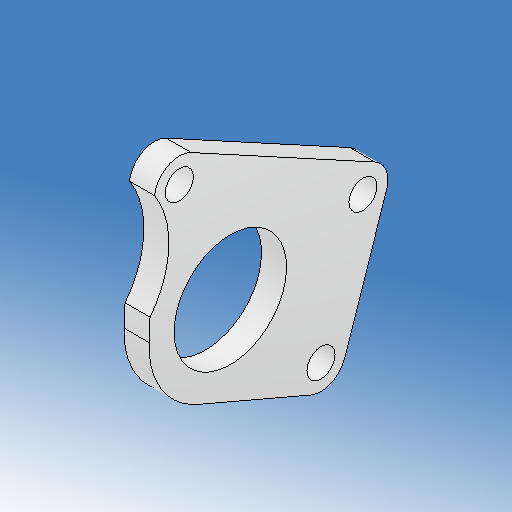
# Autodesk Inventor part: OuterDriveRail
Saved by Autodesk Inventor 2025 (Build 290162000, 162)
## iProperties
Created: 2023-02-06
Part Number: OuterDriveRail
Material: Aluminum 6061
Document SubType Name: Modeling
Designer: kumpu
Density: 2.7 g/cm^3
Appearance: Aluminum - Flat
Mass: 503.524 g
Surface Area: 633.713 cm^2
Volume: 186.49 cm^3
Author: kumpu
Autodesk Inventor part; units mm, degrees
ref_plane "YZ Plane" through (0, 0, 0) normal (1, 0, 0) x (0, 1, 0)
ref_plane "XZ Plane" through (0, 0, 0) normal (0, 1, 0) x (-1, 0, 0)
ref_plane "XY Plane" through (0, 0, 0) normal (0, 0, 1) x (1, 0, 0)
sketch "Sketch1" plane through (0, 0, 0) normal (1, 0, 0) x (0, 1, 0)
  line L0 (111.125, 190.5) -> (36.4799, 190.5)
  line L1 (36.4799, 190.5) -> (-11.1661, 102.5705)
  arc A0 (-11.1661, 102.5705) -> (-11.1661, 90.4695) centre (0, 96.52) ccw
  line L2 (-11.1661, 90.4695) -> (7.6076, 55.8231)
  arc A1 (-11.1661, 6.0505) -> (-11.1661, -6.0505) centre (0, 0) ccw
  line L3 (-11.1661, -6.0505) -> (7.6076, -40.6969)
  arc A2 (-11.1661, -90.4695) -> (-11.1661, -102.5705) centre (0, -96.52) ccw
  line L4 (-11.1661, -102.5705) -> (36.4799, -190.5)
  line L5 (36.4799, -190.5) -> (111.125, -190.5)
  line L6 (111.125, -190.5) -> (111.125, 190.5)
  circle A3 centre (64.6139, -120.5964) radius 6.35 construction
  circle A4 centre (42.5128, -176.727) radius 4.7625 construction
  line L7 (111.125, 0) -> (0, 0) construction
  circle A5 centre (0, 96.52) radius 2.4892 construction
  circle A6 centre (0, 0) radius 2.4892 construction
  circle A7 centre (0, -96.52) radius 2.4892 construction
  line L8 (-11.1661, 6.0505) -> (7.6076, 40.6969)
  arc A8 (7.6076, 40.6969) -> (7.6076, 55.8231) centre (-6.35, 48.26) ccw
  line L9 (-11.1661, -90.4695) -> (7.6076, -55.8231)
  arc A9 (7.6076, -55.8231) -> (7.6076, -40.6969) centre (-6.35, -48.26) ccw
  line L10 (-6.35, -48.26) -> (-6.35, 48.26) construction
  line L11 (-6.35, 0) -> (0, 0) construction
  circle A10 centre (0, 96.52) radius 3.175
  circle A11 centre (0, 0) radius 3.175
  circle A12 centre (0, -96.52) radius 3.175
  circle A13 centre (46.0375, 122.682) radius 3.5687 construction
  circle A14 centre (20.6375, 122.682) radius 3.5687 construction
  circle A15 centre (46.0375, 122.682) radius 3.175
  circle A16 centre (20.6375, 122.682) radius 3.175
  circle A17 centre (100.0125, -94.6341) radius 3.175
  circle A18 centre (74.6125, -94.6341) radius 3.175
  line L12 (0, 96.52) -> (-12.7, 96.52) construction
  circle A19 centre (60.325, -101.6) radius 3.5687 construction
  circle A20 centre (80.899, -155.6385) radius 12.0396 construction
  line L13 (30.099, -178.7242) -> (30.099, -155.6385)
  arc A21 (111.125, -114.8092) -> (30.099, -155.6385) centre (80.899, -155.6385) ccw
  circle A22 centre (60.325, -101.6) radius 3.175
  circle A23 centre (41.275, 177.125) radius 20.6375
  circle A24 centre (41.275, 177.125) radius 26.9875
  circle A25 centre (41.275, 177.125) radius 25.4 construction
  circle A26 centre (85.725, 107.3629) radius 7.9375
  line L14 (-12.7, 190.5) -> (-12.7, -193.5034) construction
  circle A27 centre (85.725, 107.3629) radius 17.78 construction
  circle A28 centre (79.375, 147.5038) radius 22.86 construction
  circle A29 centre (79.375, 147.5038) radius 14.2875
  circle A30 centre (66.675, 254) radius 58.7375 construction
  circle A31 centre (66.675, -254) radius 58.7375 construction
  circle A32 centre (80.899, -155.6385) radius 47.527 construction
  circle A33 centre (100.0125, -94.6341) radius 6.35 construction
  circle A34 centre (74.6125, -94.6341) radius 6.35 construction
  circle A35 centre (17.4625, -131.1466) radius 3.175
  circle A36 centre (17.4625, -131.1466) radius 6.35 construction
  line L15 (9.525, 127) -> (-15.875, 127) construction
  line L16 (-15.875, 127) -> (-15.875, -177.8) construction
  line L17 (-15.875, -177.8) -> (9.525, -177.8) construction
  line L18 (9.525, -177.8) -> (9.525, 127) construction
  circle A37 centre (103.1875, 79.2324) radius 3.175
  circle A38 centre (103.1875, 79.2324) radius 6.35 construction
  circle A39 centre (71.4375, 79.2324) radius 3.175
  circle A40 centre (71.4375, 79.2324) radius 6.35 construction
  line L19 (110.475, 71.2949) -> (60.975, 71.2949) construction
  line L20 (60.975, 71.2949) -> (60.975, -72.4091) construction
  line L21 (60.975, -72.4091) -> (110.475, -72.4091) construction
  line L22 (110.475, -72.4091) -> (110.475, 71.2949) construction
  line L23 (59.675, 71.2949) -> (10.175, 71.2949) construction
  line L24 (10.175, 71.2949) -> (10.175, -72.4091) construction
  line L25 (10.175, -72.4091) -> (59.675, -72.4091) construction
  line L26 (59.675, -72.4091) -> (59.675, 71.2949) construction
  circle A41 centre (99.3625, 31.9249) radius 2.0193
  circle A42 centre (99.3625, 57.3249) radius 2.0193
  circle A43 centre (73.9625, 31.9249) radius 2.0193
  circle A44 centre (73.9625, 57.3249) radius 2.0193
  circle A45 centre (48.5625, -58.4391) radius 2.0193
  circle A46 centre (48.5625, -33.0391) radius 2.0193
  circle A47 centre (23.1625, -58.4391) radius 2.0193
  circle A48 centre (23.1625, -33.0391) radius 2.0193
  line L27 (85.725, 107.3629) -> (85.725, 71.2949) construction
  line L28 (34.925, -72.4091) -> (34.925, -108.4771) construction
  circle A49 centre (-7.9375, -170.18) radius 12 construction
  line L29 (30.099, -178.7242) -> (30.099, -190.5)
  line L30 (30.099, -190.5) -> (5.0625, -190.5)
  line L31 (5.0625, -190.5) -> (5.0625, -132.5199)
  line L32 (36.4799, -190.5) -> (30.099, -190.5)
  circle A50 centre (-7.9375, -170.18) radius 13 construction
  line L33 (111.125, -104.8385) -> (80.899, -104.8385)
  line L34 (111.125, 190.5) -> (46.6374, 203.5744)
  line L35 (-8.7101, 107.103) -> (15.4999, 185.1231)
  circle A51 centre (34.925, -108.4771) radius 17.78 construction
  circle A52 centre (41.275, 177.125) radius 22.225 construction
  circle A53 centre (34.925, -108.4771) radius 7.9375
  circle A54 centre (41.275, 177.125) radius 14.2875
  point P0 (45.9508, 203.7044)
  point P1 (15.9875, 186.5519)
  point P2 (64.715, 190.5)
  point P3 (20.1393, 160.3438)
  dimension "d2" = 15.875
  dimension "d3" = 6.35
  dimension "d4" = 96.52
  dimension "d8" = 6.35
  dimension "d9" = 381
  dimension "d12" = 12.7
  dimension "d14" = 50.8
  dimension "d60" = 41.275
  dimension "d61" = 6.35
  dimension "d62" = 50.8
  dimension "d63" = 15.875
  dimension "d64" = 25.4
  dimension "d66" = 123.825
  dimension "d67" = 35.56
  dimension "d68" = 45.72
  dimension "d69" = 28.575
  dimension "d70" = 31.75
  dimension "d71" = 117.475
  dimension "d72" = 117.475
  dimension "d73" = 95.054
  dimension "d74" = 14.224
  dimension "d75" = 98.3615
  dimension "d76" = 63.5
  dimension "d77" = 44.45
  dimension "d78" = 63.5
  dimension "d79" = 12.7
  dimension "d80" = 12.7
  dimension "d81" = 25.4
  dimension "d82" = 25.4
  dimension "d83" = 304.8
  dimension "d84" = 9.525
  dimension "d89" = 31.75
  dimension "d90" = 12.7
  dimension "d91" = 4.0386
  dimension "d94" = 25.4
  dimension "d97" = 25.4
  dimension "d100" = 4.0386
  dimension "d103" = 25.4
  dimension "d106" = 25.4
  dimension "d109" = 143.704
  dimension "d110" = 143.704
  dimension "d111" = 49.5
  dimension "d112" = 49.5
  dimension "d113" = 13.97
  dimension "d114" = 11.1125
  dimension "d115" = 13.97
  dimension "d116" = 11.1125
  dimension "d117" = 50.038
  dimension "d119" = 7.9375
  dimension "d120" = 7.9375
  dimension "d121" = 11.1125
  dimension "d122" = 22.225
  dimension "d123" = 24
  dimension "d124" = 17.4625
  dimension "d125" = 7.62
  dimension "d127" = 26
  dimension "d128" = 7.9375
  dimension "d164" = 44.45
  dimension "d165" = 69.85
  dimension "d167" = 36.5125
  dimension "d169" = 50.038
  dimension "d170" = 47.1614
  dimension "d171" = 28.575
  constraints: 72 end point, 48 centre point, 22 coincident, 19 tangent, 18 point on circle, 16 equal radius, 10 horizontal, 8 vertical, 7 perpendicular, 6 parallel, 6 point on line, 4 midpoint, 2 horizontal alignment, 1 concentric, 1 equal length, 1 vertical alignment, 17 other
  measures "d2" radius of A8
  measures "d3" distance from line of L7.end L10
  measures "d4" distance of L10.start L10.end
  measures "d8" diameter of A10
  measures "d9" distance of L5.end L0.start
  measures "d12" radius of A0
  measures "d14" radius of A21
  measures "d60" diameter of A23
  measures "d61" radial gap between concentric circles of A23 A24
  measures "d62" diameter of A25
  measures "d63" diameter of A26
  measures "d64" distance from line of L6 A26.centre
  measures "d66" distance between parallel lines of L14 L6
  measures "d67" diameter of A27
  measures "d68" diameter of A28
  measures "d69" diameter of A29
  measures "d70" distance from line of L6 A29.centre
  measures "d71" diameter of A30
  measures "d72" diameter of A31
  measures "d73" diameter of A32
  measures "d74" horizontal distance of A31.centre A32.centre
  measures "d75" vertical distance of A31.centre A32.centre
  measures "d76" distance from line of L0 A30.centre
  measures "d77" distance from line of A30.centre L6
  measures "d78" distance from line of A31.centre L5
  measures "d79" diameter of A33
  measures "d80" diameter of A34
  measures "d81" distance of A18.centre A17.centre
  measures "d82" distance of L17.end L16.end
  measures "d83" distance of L16.end L15.end
  measures "d84" distance from line of A0.centre L18
  measures "d89" distance of A40.centre A37.centre
  measures "d90" vertical distance of L17.end L5.end
  measures "d91" diameter of A41
  measures "d94" distance of A41.centre A42.centre
  measures "d97" distance of A41.centre A43.centre
  measures "d100" diameter of A45
  measures "d103" distance of A45.centre A46.centre
  measures "d106" distance of A45.centre A47.centre
  measures "d109" distance of L25.end L23.start
  measures "d110" distance of L21.end L19.start
  measures "d111" distance of L23.start L23.end
  measures "d112" distance of L20.end L21.end
  measures "d113" distance from line of A42.centre L19
  measures "d114" distance from line of L22 A42.centre
  measures "d115" distance from line of L25 A45.centre
  measures "d116" distance from line of L26 A46.centre
  measures "d117" vertical distance of A44.centre A26.centre
  measures "d119" distance from line of L6 A37.centre
  measures "d120" distance from line of L19 A37.centre
  measures "d121" distance from line of A33.centre L6
  measures "d122" distance from line of A17.centre L21
  measures "d123" diameter of A49
  measures "d124" distance from line of A49.centre L18
  measures "d125" distance from line of L17 A49.centre
  measures "d127" diameter of A50
  measures "d128" distance from line of L18 A35.centre
  measures "d164" diameter of A52
  measures "d165" distance from line of A23.centre L6
  measures "d167" vertical distance of A35.centre A18.centre
  measures "d169" vertical distance of L28.end A47.centre
  measures "d170" vertical distance of A32.centre L28.end
  measures "d171" diameter of A54
extrude "Extrusion1" [suppressed]
sketch "Sketch2" plane through (12.7, 0, 0) normal (1, 0, 0) x (0, 0, -1)
  line L0 (-90.4695, -11.1661) -> (-55.8231, 7.6076) construction
  line L1 (-40.6969, 7.6076) -> (-6.0505, -11.1661) construction
  line L2 (6.0505, -11.1661) -> (40.6969, 7.6076) construction
  line L3 (55.8231, 7.6076) -> (90.4695, -11.1661) construction
  line L4 (-107.103, -8.7101) -> (-102.5705, -11.1661) construction
  arc A0 (104.8385, 80.899) -> (155.6385, 30.099) centre (155.6385, 80.899) ccw construction
  line L5 (102.5705, -11.1661) -> (178.7242, 30.099) construction
  circle A1 centre (-190.5, 111.125) radius 3.9688 construction
  circle A2 centre (-146.05, 85.725) radius 7.9375 construction
  circle A3 centre (-146.05, 85.725) radius 3.9688 construction
  circle A4 centre (-152.4, 60.325) radius 3.175 construction
  circle A5 centre (-152.4, 60.325) radius 3.9688 construction
  circle A6 centre (-122.682, 46.0375) radius 3.175 construction
  circle A7 centre (-122.682, 46.0375) radius 3.9688 construction
  circle A8 centre (-122.682, 20.6375) radius 3.175 construction
  circle A9 centre (-122.682, 20.6375) radius 3.9688 construction
  circle A10 centre (-96.52, 0) radius 3.175 construction
  circle A11 centre (-96.52, 0) radius 3.9688 construction
  circle A12 centre (0, 0) radius 3.175 construction
  circle A13 centre (0, 0) radius 3.9688 construction
  circle A14 centre (96.52, 0) radius 3.175 construction
  circle A15 centre (96.52, 0) radius 3.9688 construction
  circle A16 centre (101.6, 60.325) radius 3.175 construction
  circle A17 centre (101.6, 60.325) radius 3.9688 construction
  circle A18 centre (92.075, 34.925) radius 7.9375 construction
  circle A19 centre (92.075, 34.925) radius 3.9688 construction
  circle A20 centre (94.6341, 74.6125) radius 3.175 construction
  circle A21 centre (94.6341, 74.6125) radius 3.9688 construction
  circle A22 centre (94.6341, 100.0125) radius 3.175 construction
  circle A23 centre (94.6341, 100.0125) radius 3.9688 construction
  line L6 (-190.5, 111.125) -> (-146.05, 85.725) construction
  line L7 (-146.05, 85.725) -> (-152.4, 60.325) construction
  line L8 (-152.4, 60.325) -> (-122.682, 46.0375) construction
  line L9 (-152.4, 60.325) -> (-190.5, 111.125) construction
  line L10 (-122.682, 20.6375) -> (-152.4, 60.325) construction
  line L11 (-122.682, 20.6375) -> (-96.52, 0) construction
  line L12 (94.6341, 100.0125) -> (94.6341, 74.6125) construction
  line L13 (94.6341, 74.6125) -> (101.6, 60.325) construction
  line L14 (101.6, 60.325) -> (92.075, 34.925) construction
  line L15 (92.075, 34.925) -> (96.52, 0) construction
  line L16 (96.52, 0) -> (101.6, 60.325) construction
  line L17 (92.075, 34.925) -> (94.6341, 74.6125) construction
  line L18 (101.6, 60.325) -> (94.6341, 100.0125) construction
  line L19 (-122.682, 46.0375) -> (-96.52, 0) construction
  line L20 (104.8385, 111.125) -> (104.8385, 111.125) construction
  line L21 (-146.05, 85.725) -> (-106.0133, 111.125) construction
  circle A24 centre (-122.682, 46.0375) radius 3.175 projected
  line L22 (-146.05, 85.725) -> (-106.0133, 60.325) construction
  line L23 (-106.0133, 60.325) -> (-106.0133, 111.125) construction
  line L24 (92.075, 34.925) -> (77.9653, 57.15) construction
  line L25 (77.9653, 57.15) -> (77.9653, 12.7) construction
  line L26 (77.9653, 12.7) -> (92.075, 34.925) construction
  circle A25 centre (-122.682, 20.6375) radius 3.175 construction
  line L27 (-122.682, 46.0375) -> (-122.682, 20.6375) construction
  line L28 (-122.682, 46.0375) -> (-106.0133, 60.325) construction
  line L29 (0, 0) -> (0, 111.125) construction
  line L30 (104.8385, 111.125) -> (104.8385, 111.125) construction
  line L31 (77.9653, 12.7) -> (0, 0) construction
  line L32 (96.52, 0) -> (77.9653, 12.7) construction
  circle A26 centre (-96.52, 0) radius 3.175 construction
  line L33 (-106.0133, 111.125) -> (-96.52, 0) construction
  circle A27 centre (-106.0133, 111.125) radius 3.9688 construction
  circle A28 centre (0, 111.125) radius 3.9687 construction
  line L34 (0, 0) -> (77.9653, 57.15) construction
  line L35 (77.9653, 57.15) -> (0, 111.125) construction
  line L36 (-190.5, 104.5104) -> (-190.5, -12.7)
  line L37 (-190.5, -12.7) -> (178.7242, -12.7)
  line L38 (178.7242, -12.7) -> (178.7242, 111.125)
  line L39 (178.7242, 111.125) -> (99.6211, 111.125)
  line L40 (-190.5, 111.125) -> (-190.5, 36.4799) projected
  line L41 (-175.5554, 107.1562) -> (-155.9978, 95.9805)
  line L42 (-136.5864, 96.4289) -> (-119.6775, 107.1562)
  line L43 (-119.6775, 107.1562) -> (-175.5554, 107.1562)
  line L44 (-109.982, 103.9071) -> (-109.982, 67.5429)
  line L45 (-109.982, 67.5429) -> (-132.3343, 81.7236)
  line L46 (-132.3343, 89.7264) -> (-109.982, 103.9071)
  line L47 (-152.4, 60.325) -> (-106.0133, 60.325) construction
  line L48 (-154.1502, 69.6878) -> (-153.2291, 73.3721)
  line L49 (-159.9359, 89.0888) -> (-171.5185, 95.7074)
  line L50 (-145.5286, 71.447) -> (-146.4497, 67.7627)
  line L51 (-143.7412, 64.2937) -> (-119.6775, 64.2937)
  line L52 (-119.6775, 64.2937) -> (-136.5864, 75.0211)
  line L53 (-100.5305, 93.5713) -> (-93.4492, 10.6798)
  line L54 (-54.9309, 13.9788) -> (-100.5305, 93.5713)
  line L55 (-99.1656, 107.1562) -> (-48.5749, 18.852)
  line L56 (-48.5749, 18.852) -> (-6.3001, 107.1562)
  line L57 (-6.3001, 107.1562) -> (-99.1656, 107.1562)
  line L58 (-42.0864, 14.0232) -> (-3.9688, 93.644)
  line L59 (-3.9688, 93.644) -> (-3.9688, 10.3796)
  line L60 (12.7052, 107.1562) -> (73.9966, 64.7246)
  line L61 (73.9966, 64.7246) -> (73.9966, 107.1562)
  line L62 (73.9966, 107.1562) -> (12.7052, 107.1562)
  line L63 (81.9341, 43.4938) -> (81.9341, 26.3562)
  line L64 (81.9341, 26.3562) -> (81.3681, 25.4648)
  line L65 (81.3681, 44.3852) -> (81.9341, 43.4938)
  line L66 (15.4626, 6.4136) -> (73.9966, 49.32)
  line L67 (73.9966, 49.32) -> (73.9966, 9.5477)
  line L68 (3.9688, 7.83) -> (3.9688, 103.5504)
  line L69 (3.9688, 103.5504) -> (71.1263, 57.0576)
  line L70 (71.1263, 57.0576) -> (3.9688, 7.83)
  line L71 (94.6341, 74.6125) -> (77.9653, 57.15) construction
  circle A29 centre (77.9653, 57.15) radius 3.9688 construction
  line L72 (82.9801, 56.6557) -> (89.9715, 63.98)
  line L73 (89.9715, 63.98) -> (88.8981, 47.3339)
  line L74 (88.8981, 47.3339) -> (82.9801, 56.6557)
  line L75 (97.6308, 59.41) -> (96.9187, 48.3664)
  line L76 (94.238, 66.3687) -> (97.6308, 59.41)
  line L77 (79.2423, 7.3066) -> (88.0693, 21.2105)
  arc A30 (-136.5864, 96.4289) -> (-155.9978, 95.9805) centre (-146.05, 85.725) ccw
  arc A31 (-132.3343, 81.7236) -> (-132.3343, 89.7264) centre (-146.05, 85.725) ccw
  arc A32 (-145.5286, 71.447) -> (-136.5864, 75.0211) centre (-146.05, 85.725) ccw
  arc A33 (-159.9359, 89.0888) -> (-153.2291, 73.3721) centre (-146.05, 85.725) ccw
  arc A34 (-190.5, 111.125) -> (-188.5663, 106.5622) centre (-184.15, 111.125) ccw
  arc A35 (-161.7077, 58.3023) -> (-154.7102, 51.0844) centre (-152.4, 60.325) ccw
  arc A36 (-132.1679, 21.4994) -> (-118.8104, 11.9348) centre (-122.682, 20.6375) ccw
  arc A37 (-107.3496, 2.4916) -> (-89.4091, -8.5395) centre (-96.52, 0) ccw
  arc A38 (-7.1109, -8.5395) -> (7.1109, -8.5395) centre (0, 0) ccw
  arc A39 (89.4091, -8.5395) -> (105.7359, 6.2092) centre (96.52, 0) ccw
  arc A40 (108.765, 54.049) -> (106.2813, 68.6202) centre (101.6, 60.325) ccw
  arc A41 (101.8605, 93.8073) -> (101.4363, 106.68) centre (94.6341, 100.0125) ccw
  arc A42 (-161.7077, 58.3023) -> (-188.5663, 106.5622) centre (-254.8735, 38.0558) ccw
  arc A43 (-158.047, 67.9956) -> (-171.5185, 95.7074) centre (-254.8735, 38.0558) ccw
  arc A44 (-132.1679, 21.4994) -> (-154.7102, 51.0844) centre (-159.584, 23.9903) ccw
  circle A45 centre (-152.4, 60.325) radius 3.175 projected
  arc A46 (-154.1502, 69.6878) -> (-158.047, 67.9956) centre (-152.4, 60.325) ccw
  arc A47 (-143.7412, 64.2937) -> (-146.4497, 67.7627) centre (-152.4, 60.325) ccw
  arc A48 (-107.3496, 2.4916) -> (-118.8104, 11.9348) centre (-115.4372, 4.3524) ccw
  arc A49 (-7.1109, -8.5395) -> (-89.4091, -8.5395) centre (-48.26, -57.9553) ccw
  arc A50 (89.4091, -8.5395) -> (7.1109, -8.5395) centre (48.26, -57.9553) ccw
  arc A51 (99.6211, 111.125) -> (101.4363, 106.68) centre (105.9711, 111.125) ccw
  arc A52 (101.8605, 93.8073) -> (106.2813, 68.6202) centre (114.4128, 83.029) ccw
  circle A53 centre (-48.26, 10.3187) radius 3.9688 construction
  circle A54 centre (77.9653, 12.7) radius 3.9688 construction
  arc A55 (-54.9309, 13.9788) -> (-86.0187, 3.6345) centre (-48.26, -57.9553) ccw
  arc A56 (-10.5013, 3.6345) -> (-42.0864, 14.0232) centre (-48.26, -57.9553) ccw
  arc A57 (-3.9688, 10.3796) -> (-10.5013, 3.6345) centre (0, 0) ccw
  arc A58 (-6.0505, -11.1661) -> (6.0505, -11.1661) centre (0, 0) ccw projected
  line L78 (0, 111.125) -> (-48.26, 10.3187) construction
  line L79 (-48.26, 10.3187) -> (-106.0133, 111.125) construction
  line L80 (0, 0) -> (-96.52, 0) construction
  line L81 (-48.26, 6.35) -> (-48.26, 0) construction
  arc A59 (-86.0187, 3.6345) -> (-93.4492, 10.6798) centre (-96.52, 0) ccw
  arc A60 (94.3607, 10.9007) -> (86.0187, 3.6345) centre (96.52, 0) ccw
  arc A61 (86.0187, 3.6345) -> (79.2423, 7.3066) centre (48.26, -57.9553) ccw
  arc A62 (73.9966, 9.5477) -> (15.4626, 6.4136) centre (48.26, -57.9553) ccw
  arc A63 (99.4166, 22.668) -> (102.6192, 44.5662) centre (92.075, 34.925) ccw
  arc A64 (95.8015, 48.718) -> (96.9187, 48.3664) centre (92.075, 34.925) ccw
  arc A65 (81.3681, 44.3852) -> (81.3681, 25.4648) centre (92.075, 34.925) ccw
  arc A66 (88.0693, 21.2105) -> (91.6956, 20.6425) centre (92.075, 34.925) ccw
  arc A67 (108.765, 54.049) -> (102.6192, 44.5662) centre (138.319, 28.1619) ccw
  arc A68 (99.4166, 22.668) -> (105.7359, 6.2092) centre (138.319, 28.1619) ccw
  arc A69 (94.238, 66.3687) -> (97.4162, 51.768) centre (101.6, 60.325) ccw
  arc A70 (97.4162, 51.768) -> (95.8015, 48.718) centre (138.319, 28.1619) ccw
  arc A71 (91.6956, 20.6425) -> (94.3607, 10.9007) centre (138.319, 28.1619) ccw
  line L82 (-96.52, 0) -> (-48.26, 10.3187) construction
  line L83 (0, 0) -> (-48.26, 10.3187) construction
  point P0 (69.85, 74.6125)
  point P1 (-173.2979, 46.2664)
  point P2 (114.8092, 111.125)
  point P3 (132.5199, 5.0625)
  point P4 (97.1469, 51.9051)
  point P5 (97.1024, 51.2158)
  dimension "d33" = 7.9375
  dimension "d34" = 44.45
  dimension "d35" = 50.8
  dimension "d37" = 16.6687
  dimension "d38" = 16.6687
  dimension "d39" = 14.2875
  dimension "d40" = 9.525
  dimension "d41" = 11.1125
  dimension "d42" = 6.35
  dimension "d44" = 6.35
  dimension "d46" = 14.2875
  dimension "d47" = 7.9375
  constraints: 153 end point, 80 point on circle, 61 tangent, 55 centre point, 37 equal radius, 32 coincident, 29 parallel, 12 concentric, 10 vertical, 4 horizontal, 4 perpendicular, 2 equal length, 2 point on line, 1 collinear, 1 midpoint, 6 other
  measures "d33" diameter of A1
  measures "d34" distance of L24.end L25.end
  measures "d35" distance of L22.end L21.end
  measures "d37" distance between parallel lines of L25 L12
  measures "d38" distance between parallel lines of L27 L23
  measures "d39" radius of A30
  measures "d40" radius of A35
  measures "d41" radius of A37
  measures "d42" radius of A34
  measures "d44" distance of L81.start L81.end
  measures "d46" radius of A63
  measures "d47" radial gap between concentric circles of A67 A70
extrude "Extrusion2" [suppressed]
delete_face "Delete Face1" [suppressed]
fillet "Fillet2" [suppressed]
fillet "Fillet3" [suppressed]
fillet "Fillet4" [suppressed]
sketch "Sketch3" plane through (0, 111.125, 190.5) normal (0, 1, 0) x (1, 0, 0)
  circle A0 centre (69.85, 18.9559) radius 3.175
  circle A1 centre (69.85, 87.1601) radius 3.175
  circle A2 centre (69.85, 190.5) radius 3.175
  circle A3 centre (69.85, 274.2219) radius 3.175
  line L0 (63.5, 381) -> (63.5, 0)
  line L1 (12.7, 0) -> (12.7, 1.9337) projected
  line L2 (63.5, 0) -> (12.7, 0)
  line L3 (12.7, 0) -> (38.1, 0)
  line L4 (38.1, 22.1309) -> (38.1, 0)
  circle A4 centre (6.35, 18.9559) radius 3.175
  circle A5 centre (6.35, 87.1601) radius 3.175
  circle A6 centre (6.35, 190.5) radius 3.175
  circle A7 centre (6.35, 12.5087) radius 3.175
  line L5 (12.7, 19.3349) -> (12.7, 20.9224) projected
  circle A8 centre (6.35, 248.6025) radius 3.175
  point P0 (0, 190.5)
  point P1 (12.7, 20.1348)
  point P2 (12.7, 20.1287)
  point P3 (12.7, 239.7125)
  dimension "d51" = 6.35
  dimension "d52" = 7.62
  dimension "d53" = 6.35
  dimension "d54" = 8.89
  constraints: 9 centre point, 8 end point, 3 symmetric about line, 2 midpoint, 1 horizontal, 1 perpendicular, 1 vertical, 13 other
  measures "d51" diameter of A7
  measures "d52" vertical distance of point (12.7, 20.129) A7.centre
  measures "d53" diameter of A8
  measures "d54" vertical distance of A8.centre point (12.7, 239.712)
extrude "Extrusion3" [suppressed]
extrude "Extrusion4" [suppressed]
fillet "Fillet5" [suppressed]
fillet "Fillet6" [suppressed]
sketch "Sketch4" plane through (12.7, 0, 0) normal (1, 0, 0) x (0, 0, -1)
  line L0 (177.8, 9.525) -> (-127, 9.525) construction
  line L1 (-127, 9.525) -> (-127, -15.875) construction
  line L2 (-127, -15.875) -> (177.8, -15.875) construction
  line L3 (-190.5, -12.7) -> (193.5034, -12.7) construction
  line L4 (177.8, -15.875) -> (177.8, 9.525) construction
  line L5 (-151.384, 167.5964) -> (215.7494, 167.5964) construction
  line L6 (215.7494, 167.5964) -> (215.7494, 66.675) construction
  line L7 (215.7494, 66.675) -> (-151.384, 66.675) construction
  line L8 (-151.384, 66.675) -> (-151.384, 167.5964) construction
  circle A0 centre (155.6385, 99.949) radius 47.527 construction
  circle A1 centre (92.075, 34.925) radius 7.9375 projected
  circle A2 centre (92.075, 34.925) radius 22.225 construction
  line L9 (-138.684, 66.675) -> (64.516, 66.675) construction
  line L10 (64.516, 66.675) -> (64.516, 15.875) construction
  line L11 (64.516, 15.875) -> (-138.684, 15.875) construction
  line L12 (-138.684, 15.875) -> (-138.684, 66.675) construction
  circle A3 centre (-147.5038, 79.375) radius 14.2875 construction
  circle A4 centre (-177.125, 41.275) radius 20.6375 construction
  circle A5 centre (-107.3629, 85.725) radius 7.9375 construction
  circle A6 centre (-147.5038, 79.375) radius 22.86 construction
  circle A7 centre (-107.3629, 85.725) radius 17.78 construction
  circle A8 centre (-177.125, 41.275) radius 25.4 construction
  circle A9 centre (-75.184, 53.975) radius 3.175
  circle A10 centre (-100.584, 28.575) radius 3.175
  circle A11 centre (-62.484, 28.575) radius 3.175
  circle A12 centre (-37.084, 53.975) radius 3.175
  circle A13 centre (-24.384, 28.575) radius 3.175
  circle A14 centre (1.016, 53.975) radius 3.175
  circle A15 centre (-122.682, 46.0375) radius 3.175 construction
  circle A16 centre (-122.682, 20.6375) radius 3.175 construction
  circle A17 centre (13.716, 28.575) radius 3.175
  point P0 (0, 0)
  point P1 (155.6385, 80.899)
  dimension "d130" = 82.55
  dimension "d131" = 367.1334
  dimension "d132" = 100.9214
  dimension "d133" = 60.1109
  dimension "d134" = 95.054
  dimension "d135" = 33.274
  dimension "d136" = 44.45
  dimension "d137" = 203.2
  dimension "d138" = 12.7
  dimension "d139" = 35.56
  dimension "d140" = 45.72
  dimension "d141" = 50.8
  dimension "d142" = 50.8
  dimension "d143" = 6.35
  dimension "d145" = 38.1
  dimension "d146" = 76.2
  dimension "d147" = 38.1
  dimension "d148" = 76.2
  dimension "d149" = 25.4
  dimension "d150" = 25.4
  dimension "d151" = 12.7
  dimension "d152" = 38.1
  dimension "d153" = 114.3
  constraints: 16 end point, 12 centre point, 6 equal radius, 4 coincident, 4 horizontal alignment, 4 parallel, 2 horizontal, 2 perpendicular, 1 point on line, 1 vertical alignment
  measures "d130" distance between parallel lines of L2 L7
  measures "d131" distance of L5.start L5.end
  measures "d132" distance of L5.end L6.end
  measures "d133" distance from line of L6 A0.centre
  measures "d134" diameter of A0
  measures "d135" distance from line of L7 A0.centre
  measures "d136" diameter of A2
  measures "d137" distance between parallel lines of L10 L12
  measures "d138" distance between parallel lines of L12 L8
  measures "d139" diameter of A7
  measures "d140" diameter of A6
  measures "d141" diameter of A8
  measures "d142" distance of L9.end L10.end
  measures "d143" diameter of A9
  measures "d145" distance of A11.centre A10.centre
  measures "d146" distance of A13.centre A10.centre
  measures "d147" distance of A12.centre A9.centre
  measures "d148" distance of A14.centre A9.centre
  measures "d149" horizontal distance of A9.centre A10.centre
  measures "d150" horizontal distance of A10.centre A9.centre
  measures "d151" distance from line of L11 A10.centre
  measures "d152" distance from line of A10.centre L12
  measures "d153" distance of A17.centre A10.centre
extrude "Extrusion5" [suppressed]
sketch "Sketch6" plane through (12.7, 0, 0) normal (1, 0, 0) x (0, 0, -1)
  circle A0 centre (-190.0765, 73.025) radius 3.175
  circle A1 centre (-143.4281, 47.625) radius 3.175
  circle A2 centre (-154.0893, 15.875) radius 3.175
  circle A3 centre (-190.0765, 73.025) radius 6.35 construction
  circle A4 centre (-143.4281, 47.625) radius 6.35 construction
  circle A5 centre (-154.0893, 15.875) radius 6.35 construction
  circle A6 centre (-177.125, 41.275) radius 14.2875 construction
  circle A7 centre (-177.125, 41.275) radius 34.29 construction
  line L0 (104.8385, 111.125) -> (-190.5, 111.125) construction
  circle A8 centre (-147.5038, 79.375) radius 14.2875 construction
  circle A9 centre (-147.5038, 79.375) radius 22.86 construction
  circle A10 centre (-177.125, 41.275) radius 25.4 construction
  line L1 (-190.0765, 73.025) -> (-154.0893, 15.875) construction
  line L2 (-154.0893, 15.875) -> (-143.4281, 47.625) construction
  line L3 (-143.4281, 47.625) -> (-190.0765, 73.025) construction
  point P0 (0, 0)
  dimension "d172" = 6.35
  dimension "d173" = 12.7
  dimension "d176" = 63.5
  dimension "d177" = 95.25
  dimension "d180" = 68.58
  dimension "d181" = 45.72
  dimension "d182" = 38.1
  constraints: 7 centre point, 6 end point, 4 coincident, 4 equal radius, 3 point on circle
  measures "d172" diameter of A0
  measures "d173" diameter of A3
  measures "d176" distance from line of L0 A1.centre
  measures "d177" distance from line of L0 A2.centre
  measures "d180" diameter of A7
  measures "d181" diameter of A9
  measures "d182" distance from line of L0 A0.centre
extrude "Extrusion6" [suppressed]
sketch "Sketch7" plane through (12.7, 0, 0) normal (1, 0, 0) x (0, 0, -1)
  circle A0 centre (-107.3629, 85.725) radius 7.9375 projected
  circle A1 centre (-107.3629, 85.725) radius 12.6996 construction
  circle A2 centre (-116.3429, 94.705) radius 1
  circle A3 centre (-116.3429, 76.745) radius 1
  circle A4 centre (-98.3829, 76.745) radius 1
  circle A5 centre (-98.3829, 94.705) radius 1
  circle A6 centre (108.4771, 34.925) radius 7.9375 construction
  circle A7 centre (108.4771, 34.925) radius 12.6996 construction
  circle A8 centre (99.4971, 43.905) radius 1
  circle A9 centre (99.4971, 25.945) radius 1
  circle A10 centre (117.4571, 25.945) radius 1
  circle A11 centre (117.4571, 43.905) radius 1
  point P0 (0, 0)
  dimension "d183" = 25.3993
  dimension "d184" = 8.98
  dimension "d185" = 2
  dimension "d188" = 360
  dimension "d190" = 2
  dimension "d191" = 8.98
  dimension "d194" = 360
  constraints: 8 centre point, 2 coincident, 24 other
  measures "d184" horizontal distance of A0.centre A2.centre
  measures "d185" diameter of A2
  measures "d190" diameter of A8
  measures "d191" horizontal distance of A6.centre A8.centre
extrude "Extrusion7" [suppressed]
sketch "Sketch8" plane through (0, 0, 0) normal (1, 0, 0) x (0, 1, 0)
  circle A0 centre (41.275, 177.125) radius 14.2875 projected
  circle A1 centre (73.025, 190.0765) radius 3.175 projected
  circle A2 centre (41.275, 177.125) radius 14.2875 construction
  circle A3 centre (15.875, 154.0893) radius 3.175 projected
  circle A4 centre (41.275, 177.125) radius 34.29 construction
  circle A5 centre (47.625, 143.4281) radius 3.175 projected
  circle A6 centre (73.025, 190.0765) radius 6.35 construction
  circle A7 centre (47.625, 143.4281) radius 6.35 construction
  circle A8 centre (15.875, 154.0893) radius 6.35 construction
  circle A9 centre (41.275, 177.125) radius 20.6375 construction
  line L0 (73.2945, 196.4208) -> (42.151, 197.7439)
  line L1 (22.3021, 185.2451) -> (10.0372, 156.5878)
  line L2 (13.8537, 148.0696) -> (45.6037, 137.4084)
  line L3 (53.2019, 140.3915) -> (78.6019, 187.0399)
  arc A10 (78.6019, 187.0399) -> (73.2945, 196.4208) centre (73.025, 190.0765) ccw
  arc A11 (42.151, 197.7439) -> (22.3021, 185.2451) centre (41.275, 177.125) ccw
  arc A12 (10.0372, 156.5878) -> (13.8537, 148.0696) centre (15.875, 154.0893) ccw
  arc A13 (45.0971, 137.6029) -> (53.2019, 140.3915) centre (47.625, 143.4281) ccw
  circle A14 centre (73.025, 190.0765) radius 3.5719
  circle A15 centre (47.625, 143.4281) radius 3.5719
  circle A16 centre (15.875, 154.0893) radius 3.5719
  point P0 (0, 0)
  dimension "d198" = 3.175
  dimension "d199" = 6.35
  dimension "d202" = 7.1437
  dimension "d203" = 7.1437
  dimension "d204" = 7.1437
  constraints: 17 point on circle, 11 centre point, 8 end point, 8 tangent, 7 coincident, 3 equal radius
  measures "d198" radial gap between concentric circles of A1 A6
  measures "d199" radial gap between concentric circles of A0 A9
  measures "d202" diameter of A14
  measures "d203" diameter of A15
  measures "d204" diameter of A16
extrude "Extrusion8" add sketch "Sketch8" along normal blind 6.35 contours A10 L3 A13 L2 A12 L1 A11 L0
sketch "Sketch9" plane through (6.35, 0, 0) normal (1, 0, 0) x (0, 0, -1)
  arc A0 (-197.5113, 47.625) -> (-196.3978, 73.8357) centre (-215.2693, 61.5084) ccw
  circle A1 centre (-177.125, 41.275) radius 14.2875 projected
  circle A2 centre (-190.0765, 73.025) radius 3.5719 projected
  circle A3 centre (-190.0765, 73.025) radius 5.1594
  circle A4 centre (-177.125, 41.275) radius 20.6375
  line L0 (-196.3978, 73.8357) -> (-197.5113, 47.625)
  line L1 (-196.4208, 73.2945) -> (-197.7439, 42.151) projected
  point P0 (0, 0)
  dimension "d205" = 1.5875
  dimension "d206" = 6.35
  dimension "d213" = 6.35
  constraints: 3 centre point, 2 end point, 2 point on circle, 2 point on line, 2 tangent
  measures "d205" radial gap between concentric circles of A2 A3
  measures "d206" radial gap between concentric circles of A1 A4
  measures "d213" vertical distance of A1.centre L0.end
extrude "Extrusion9" cut sketch "Sketch9" against normal blind 25.4 contours L0 A0
body "Solid1"
